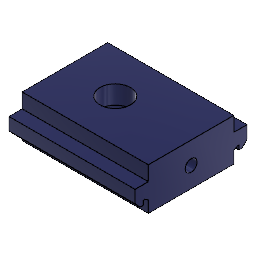
3-Pulley_Bearing_Mount_V2 v3 (Autodesk Fusion 360 design; units mm, degrees)
Autodesk Fusion 360 part; units mm, degrees
sketch "Main Profile" plane through (0, 0, 0) normal (1, 0, 0) x (0, 1, 0)
  line L0 (-19.75, -9.75) -> (19.75, -9.75)
  line L1 (19.75, -9.75) -> (19.75, 9.75)
  line L2 (19.75, 9.75) -> (-19.75, 9.75)
  line L3 (-19.75, 9.75) -> (-19.75, -9.75)
  line L4 (-19.75, -9.75) -> (19.75, 9.75) construction
  line L5 (19.75, -9.75) -> (-19.75, 9.75) construction
  line L6 (-19.75, 3) -> (-25.85, 3)
  line L7 (-25.85, 3) -> (-25.85, -2.8)
  line L8 (-25.85, -2.8) -> (-23.5187, -5.3)
  line L9 (-23.5187, -5.3) -> (-22.05, -5.3)
  line L10 (-22.05, -5.3) -> (-22.05, -3.3)
  line L11 (-22.05, -3.3) -> (-21.35, -3.3)
  line L12 (-21.35, -3.3) -> (-19.75, -4.2238)
  line L13 (0, 9.75) -> (0, -9.75) construction
  line L14 (19.75, 3) -> (25.85, 3)
  line L15 (25.85, 3) -> (25.85, -2.8)
  line L16 (25.85, -2.8) -> (23.5187, -5.3)
  line L17 (23.5187, -5.3) -> (22.05, -5.3)
  line L18 (22.05, -5.3) -> (22.05, -3.3)
  line L19 (22.05, -3.3) -> (21.35, -3.3)
  line L20 (21.35, -3.3) -> (19.75, -4.2238)
  circle A0 centre (0, -0.4) radius 2.75
  dimension "d1" = 39.5
  dimension "d2" = 19.5
  dimension "d3" = 6.1
  dimension "d4" = 6.75
  dimension "d5" = 8.3
  dimension "d6" = 43
  dimension "d7" = 2.5
  dimension "d8" = 120
  dimension "d9" = 3.8
  dimension "d10" = 2
  dimension "d11" = 1.6
  dimension "d12" = 5.5
  dimension "d13" = 0.4
  constraint perpendicular L0 L1
  constraint parallel L0 L2
  constraint parallel L1 L3
  constraint horizontal L0
  constraint coincident L4 origin
  constraint coincident L5 origin
  constraint coincident L3 L6.start
  constraint perpendicular L3 L6
  constraint perpendicular L6 L7
  constraint perpendicular L3 L9
  constraint perpendicular L9 L10
  constraint perpendicular L3 L11
  constraint coincident L3 L12.end
  constraint midpoint L2 L13.start
  constraint midpoint L0 L13.end
  constraint symmetric L6.start L13 L14.start
  constraint symmetric L6.end L13 L14.end
  constraint symmetric L7.end L13 L15.end
  constraint symmetric L8.end L13 L16.end
  constraint symmetric L9.end L13 L17.end
  constraint symmetric L10.end L13 L18.end
  constraint symmetric L11.end L13 L19.end
  constraint symmetric L12.end L13 L20.end
  constraint coincident L13 A0.centre
  measures "d1" distance of L1.end L2.end
  measures "d2" distance of L0.end L1.end
  measures "d3" distance of L3 L7
  measures "d4" distance of L2 L6
  measures "d5" distance of L6 L9
  measures "d6" angle of L7 L8
  measures "d7" vertical distance of L7.end L8.end
  measures "d8" angle of L3 L12
  measures "d9" distance of L7 L10
  measures "d10" distance of L9 L11
  measures "d11" horizontal distance of L11.end L12.end
  measures "d12" diameter of A0
  measures "d13" distance of origin A0.centre
extrude "Extrude1" add sketch "Main Profile" against normal blind 58.25 contours L0 L1 L2 L3 | L3 L6 L7 L8 L9 L10 L11 L12 | L1 L14 L15 L16 L17 L18 L19 L20 | A0
sketch "Side" plane through (0, 0, -9.75) normal (0, 0, -1) x (1, 0, 0)
  line L0 (0, -19.75) -> (0, 19.75)
  line L1 (0, 19.75) -> (-58.25, 19.75)
  line L2 (-58.25, 19.75) -> (-58.25, -19.75)
  line L3 (-58.25, -19.75) -> (0, -19.75)
  circle A0 centre (-35, 0) radius 17.75
  circle A1 centre (-35, 0) radius 7
  line L4 (-10.25, -4.25) -> (-5.75, -4.25)
  line L5 (-5.75, -4.25) -> (-5.75, 4.25)
  line L6 (-5.75, 4.25) -> (-10.25, 4.25)
  line L7 (-10.25, 4.25) -> (-10.25, -4.25)
  line L8 (-10.25, -4.25) -> (-5.75, 4.25) construction
  line L9 (-5.75, -4.25) -> (-10.25, 4.25) construction
  point P0 (-8, 0)
  dimension "d16" = 35.5
  dimension "d17" = 35
  dimension "d18" = 14
  dimension "d19" = 8.5
  dimension "d20" = 4.5
  dimension "d21" = 5.75
  constraint horizontal origin A0.centre
  constraint concentric A0 A1
  constraint perpendicular L4 L5
  constraint parallel L4 L6
  constraint parallel L5 L7
  constraint horizontal L4
  constraint coincident L8 P0
  constraint coincident L9 P0
  constraint horizontal origin P0
  measures "d16" diameter of A0
  measures "d17" distance of L0 A0.centre
  measures "d18" diameter of A1
  measures "d19" distance of L4.end L5.end
  measures "d20" distance of L5.end L6.end
  measures "d21" distance of origin L5
extrude "Extrude2" cut sketch "Side" against normal blind 13.5 contours L4 L5 L6 L7
extrude "Extrude3" cut sketch "Side" against normal blind 40 contours A1
extrude "Extrude4" cut sketch "Side" against normal blind 10.85 contours A0
extrude "Extrude5" cut sketch "Main Profile" against normal blind 15.75 contours A0
extrude "Extrude6" cut 1 faces at (-20.8994, 0.8818, 1.1) along direction (0, 0, 1) blind 0.15
named bodies: "3-Pulley_Bearing_Mount_V2"
